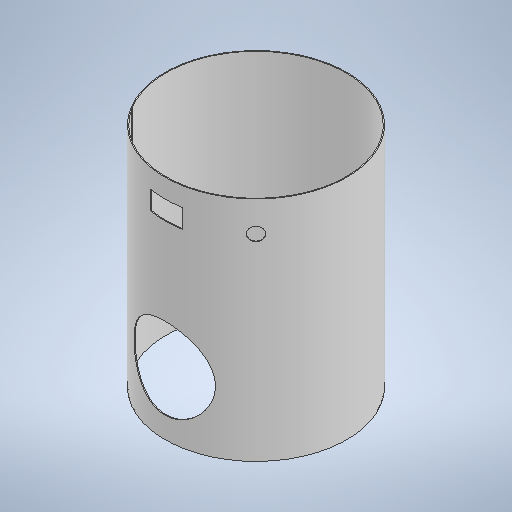
# Autodesk Inventor part: PRS 000 Filter1200 MAIN Shell
Saved by Autodesk Inventor 2026.2 (Build 302298000, 298)
## iProperties
Created: 2025-02-11
Part Number: PRS 000 Filter1200 MAIN Shell
Material: Steel
Document SubType Name: Sheet Metal
Designer: pokla
Mass: 197479 g
Surface Area: 84554.1 cm^2
Volume: 25156.5 cm^3
Density: 7.85 g/cm^3
Flat Pattern Width: 150 cm
Flat Pattern Length: 374.776 cm
Flat Pattern Area: 56216.4 cm^2
Sheet Metal Rule: Default_mm
Sheet Metal Width: 1500,000 mm
Sheet Metal Length: 3747,758 mm
Sheet Metal Area: 5621637,523 mm^2
Appearance: Default
Author: pokla
Autodesk Inventor part; units mm, degrees
ref_plane "YZ Plane" through (0, 0, 0) normal (1, 0, 0) x (0, 1, 0)
ref_plane "XZ Plane" through (0, 0, 0) normal (0, 1, 0) x (-1, 0, 0)
ref_plane "XY Plane" through (0, 0, 0) normal (0, 0, 1) x (1, 0, 0)
sketch "Sketch13" plane through (0, 0, 0) normal (0, 0, 1) x (1, 0, 0)
  circle A0 centre (0, 0) radius 600 construction
  line L0 (0, 0) -> (0, -600)
  line L1 (0, 0) -> (-508.8289, -317.9516)
  line L2 (0, 0) -> (424.2641, -424.2641)
  line L3 (0, 0) -> (0, -600)
  line L4 (0, 0) -> (0, -600)
  line L5 (0, 0) -> (-534.6039, -272.3943)
  arc A1 (-508.8289, -317.9516) -> (0, -600) centre (0, 0) ccw
  dimension "d53" = 1200
  dimension "d54" = 58
  dimension "d55" = 0
  dimension "d56" = 0
  dimension "d57" = 315
  dimension "d58" = 63
  constraints: 12 end point, 8 point on circle, 2 centre point, 2 coincident, 1 vertical
  measures "d53" diameter of A0
  measures "d54" angle of L0 L1
  measures "d55" distance between parallel lines of L0 L4
  measures "d56" distance between parallel lines of L0 L3
  measures "d58" angle of L0 L5
ref_plane "WeldJoint" through (0, 0, -10) normal (0.5299193, -0.8480481, 0) x (0, 0, 1)
ref_plane "Inlet_Clock_Angle_plane" through (0, 0, -10) normal (0.7071068, 0.7071068, 0) x (0, 0, 1)
ref_plane "Charging" through (0, 0, -10) normal (1, 0, 0) x (0, 0, 1)
ref_plane "Accsess" through (0, 0, -10) normal (1, 0, 0) x (0, 0, 1)
sketch "Sketch14" plane through (0, 0, -10) normal (0.5299193, -0.8480481, 0) x (0, 0, 1)
  line L0 (1510, 594) -> (10, 594)
  line L1 (10, 594) -> (10, 600)
  line L2 (10, 600) -> (1510, 600)
  line L3 (1510, 600) -> (1510, 594)
  line L4 (10, 0) -> (1510, 0)
  line L5 (10, 600) -> (-20, 600) construction
  line L6 (10, 594) -> (-20, 594) construction
  arc A0 (-20, 594) -> (-108.189, 541.1455) centre (-20, 494) ccw construction
  arc A1 (-108.189, 541.1455) -> (-240, 15) centre (876.0042, 15) ccw construction
  line L7 (-240, 15) -> (-240, 0) construction
  line L8 (10, 0) -> (-240, 0) construction
  arc A2 (-20, 600) -> (-113.4804, 543.9742) centre (-20, 494) ccw construction
  arc A3 (-113.4804, 543.9742) -> (-246, 15) centre (876.0042, 15) ccw construction
  line L9 (-246, 15) -> (-246, 0) construction
  line L10 (-240, 0) -> (-246, 0) construction
  line L11 (1510, 594) -> (1540, 594)
  line L12 (1510, 600) -> (1540, 600)
  line L13 (1510, 0) -> (1760, 0) construction
  line L14 (1766, 0) -> (1766, 15) construction
  arc A4 (1766, 15) -> (1633.4804, 543.9742) centre (643.9958, 15) ccw construction
  arc A5 (1633.4804, 543.9742) -> (1540, 600) centre (1540, 494) ccw construction
  line L15 (1760, 0) -> (1760, 15) construction
  line L16 (1760, 0) -> (1766, 0) construction
  arc A6 (1760, 15) -> (1628.189, 541.1455) centre (643.9958, 15) ccw construction
  arc A7 (1628.189, 541.1455) -> (1540, 594) centre (1540, 494) ccw construction
  line L17 (-159.0801, 530) -> (-604, 530)
  line L18 (-604, 530) -> (-604, 450)
  line L19 (-604, 450) -> (-159.0801, 450)
  line L20 (-159.0801, 450) -> (-159.0801, 530)
  line L21 (1766, 15) -> (1796, 15) construction
  line L22 (1796, 15) -> (1796, 0) construction
  line L23 (1796, 0) -> (1766, 0) construction
  line L24 (-604, 610) -> (-604, 530)
  line L25 (-604, 610) -> (-598, 610)
  line L26 (-598, 610) -> (-598, 530)
  line L27 (-115.594, 543.6036) -> (-167.5067, 431.8618)
  line L28 (-159.0801, 530) -> (-121.9139, 530)
  line L29 (-108.189, 541.1455) -> (-113.4804, 543.9742)
  line L30 (-115.594, 543.6036) -> (-115.0356, 544.8056) construction
  line L31 (-115.0356, 544.8056) -> (-113.4804, 543.9742) construction
  point P0 (10, 597)
  point P1 (-141.5503, 487.7327)
  dimension "d59" = 1500
  dimension "d60" = 6
  dimension "d61" = 1200
  dimension "d82" = 100
  dimension "d83" = 30
  dimension "d84" = 30
  dimension "d85" = 250
  dimension "d86" = 80
  dimension "d87" = 30
  dimension "d88" = 2400
  dimension "d90" = 900
  dimension "d91" = 15
  dimension "d92" = 20
  constraints: 64 end point, 18 point on circle, 13 tangent, 12 horizontal, 8 centre point, 7 perpendicular, 6 equal length, 6 point on line, 4 concentric, 4 parallel, 2 collinear, 2 equal radius, 2 midpoint, 2 vertical, 1 vertical alignment
  measures "d59" distance of L1.end L2.end
  measures "d60" distance of L0.end L1.end
  measures "d61" diameter of L2 L4
  measures "d82" radius of A0
  measures "d83" distance of L0.end L6.end
  measures "d84" diameter of L7.start L4
  measures "d85" distance of L7.end L4.start
  measures "d86" distance of L17.end L18.end
  measures "d87" distance of L14.end L21.end
  measures "d88" distance between parallel lines of L22 L18
  measures "d90" diameter of L19 L4
  measures "d91" distance of L28.end L27.start
  measures "d92" distance of L19.end L27.end
revolve "Revolution2" add sketch "Sketch14" angle 359.9 about axis through (0, 0, 0) along (0, 0, 1) contours L0 L1 L2 L3
sketch "Sketch AnglePlane_InletPipe" plane through (0, 0, -10) normal (0.7071068, 0.7071068, 0) x (0, 0, 1)
  line L0 (10, -600) -> (10, 600) projected
  line L1 (10, 0) -> (1310, 0)
  line L2 (1310, 0) -> (1310, 600)
  line L3 (1310, 600) -> (10, 600)
  line L4 (10, 600) -> (10, 0)
  point P0 (10, -134.9706)
  point P1 (10, -135.9908)
  dimension "d63" = 1200
  dimension "d64" = 90
  dimension "frd_hght" = 1300
  constraints: 8 end point, 1 collinear, 1 horizontal, 1 parallel
  measures "d63" diameter of L3 L1
  measures "d64" angle of L2 L3
  measures "frd_hght" distance of L2.end L3.end
ref_plane "InletPipe_AnglePlane" through (0, 0, 1300) normal (0.7071068, -0.7071068, 0) x (0.7071068, 0.7071068, 0)
sketch "Sketch16" plane through (0, 0, 1300) normal (0.7071068, -0.7071068, 0) x (0.7071068, 0.7071068, 0)
  circle A0 centre (0, 0) radius 45.5
  point P0 (0, -1300)
  point P1 (0, 0)
  point P2 (0, 0)
  point P3 (0, 0)
  dimension "d66" = 91
  constraints: 1 centre point, 1 coincident
  measures "d66" diameter of A0
extrude "Extrusion7" cut sketch "Sketch16" along normal through all
ref_plane "Work Plane16" through (0, 0, 0) normal (0, -1, 0) x (1, 0, 0)
sketch "Sketch17" plane through (0, 0, 0) normal (0, -1, 0) x (1, 0, 0)
  circle A0 centre (0, 408.5) radius 268.5
  line L0 (0, 140) -> (-495.5727, 140)
  point P0 (0, 0)
  dimension "d69" = 537
  dimension "d71" = 140
  constraints: 2 end point, 2 horizontal, 2 vertical alignment, 2 other
  measures "d71" distance from line of point (0, 0) L0
extrude "Extrusion8" cut sketch "Sketch17" along normal through all
sketch "Sketch19" plane through (0, 0, -10) normal (1, 0, 0) x (0, 0, 1)
  line L0 (10, 0) -> (1260, 0)
  line L1 (1260, 0) -> (1260, 600)
  line L2 (1260, 600) -> (10, 600)
  line L3 (10, 600) -> (10, 0)
  dimension "d74" = 1250
  dimension "d76" = 1200
  dimension "d77" = 90
  constraints: 8 end point, 1 horizontal, 1 parallel, 1 perpendicular
  measures "d74" distance of L1.end L2.end
  measures "d76" diameter of L2 L0
  measures "d77" angle of L2 L1
ref_plane "Work Plane18" through (0, 0, 1250) normal (0, -1, 0) x (1, 0, 0)
sketch "Sketch20" plane through (0, 0, 1250) normal (0, -1, 0) x (1, 0, 0)
  line L0 (-103.5, 0) -> (103.5, 0)
  line L1 (103.5, 0) -> (103.5, 125)
  line L2 (103.5, 125) -> (-103.5, 125)
  line L3 (-103.5, 125) -> (-103.5, 0)
  point P0 (0, -1250)
  point P1 (0, 0)
  point P2 (0, 0)
  point P3 (0, 0)
  point P4 (0, 0)
  dimension "d78" = 207
  dimension "d79" = 125
  constraints: 8 end point, 2 parallel, 1 coincident, 1 horizontal, 1 midpoint, 1 perpendicular
  measures "d78" distance of L2.end L1.end
  measures "d79" distance of L1.end L0.end
extrude "Extrusion9" cut sketch "Sketch20" along normal through all
equation "\"BendRadius\" = Thickness"
equation "\"BendReliefWidth\" = Thickness"
equation "\"BendReliefDepth\" = 0.5 * Thickness"
equation "\"CornerReliefSize\" = 4 * Thickness"
equation "\"MinimumRemnant\" = 2 * Thickness"
equation "\"TransitionRadius\" = BendRadius"
equation "\"JacobiRadiusSize\" = BendRadius"
equation "\"GapSize\" = Thickness"
equation "\"InletPipe_horisont_angle\" = 0"
equation "\"AccsessHatch_diameter\" = 535"
equation "\"AccsessHatch_ClockAngle\" = 0"
equation "\"ChargingHatch_ClockAgnle\" = 0"
equation "\"InletPipe_Clock_angle\" = 315deg"
equation "\"OutletPipe_ClockAngle\" = 63deg"
equation "\"WeldJoint_ClockAgnle\" = 58deg"
equation "\"Thickness\" = 6"
body "Solid2"
